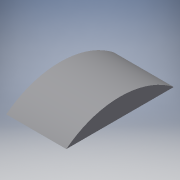
# Autodesk Inventor part: Wheel profile
Saved by Autodesk Inventor 2018 (Build 220112000, 112)
## iProperties
Created: 2018-02-21
Part Number: Wheel profile
Material: Generic
Document SubType Name: Modeling
Designer: owner
Density: 1 g/cm^3
Appearance: Default
Author: owner
Autodesk Inventor part; units mm, degrees
ref_plane "YZ Plane" through (0, 0, 0) normal (1, 0, 0) x (0, 1, 0)
ref_plane "XZ Plane" through (0, 0, 0) normal (0, 1, 0) x (-1, 0, 0)
ref_plane "XY Plane" through (0, 0, 0) normal (0, 0, 1) x (1, 0, 0)
sketch "Sketch1" plane through (0, 0, 0) normal (1, 0, 0) x (0, 1, 0)
  line L0 (0, 0) -> (0, -1181.1)
  line L1 (0, 0) -> (1181.1, 0) construction
  arc A0 (0, -1181.1) -> (0, 0) centre (-756.543, -590.55) ccw
  dimension "d0" = 1181.1
  dimension "d1" = 90
  constraints: 4 end point, 2 point on circle, 1 centre point, 1 horizontal, 1 perpendicular, 1 vertical
  measures "d0" distance of L0.start L0.end
  measures "d1" angle of L0 L1
extrude "Extrusion1" add sketch "Sketch1" along normal blind 660.4
body "Solid1"
